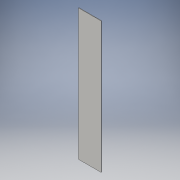
# Autodesk Inventor part: RightSidePlate
Saved by Autodesk Inventor 2016 (Build 200138000, 138)
## iProperties
Created: 2017-02-17
Part Number: RightSidePlate
Material: Generic
Document SubType Name: Modeling
Designer: RoboticsUser
Density: 1 g/cm^3
Appearance: Default
Author: RoboticsUser
Autodesk Inventor part; units mm, degrees
ref_plane "YZ Plane" through (0, 0, 0) normal (1, 0, 0) x (0, 1, 0)
ref_plane "XZ Plane" through (0, 0, 0) normal (0, 1, 0) x (-1, 0, 0)
ref_plane "XY Plane" through (0, 0, 0) normal (0, 0, 1) x (1, 0, 0)
sketch "Sketch1" plane through (0, 0, 0) normal (0, 0, 1) x (1, 0, 0)
  line L0 (0, 0) -> (76.2, 0)
  line L1 (76.2, 0) -> (76.2, 444.5)
  line L2 (76.2, 444.5) -> (0, 444.5)
  line L3 (0, 444.5) -> (0, 0)
  dimension "d0" = 76.2
  dimension "d1" = 444.5
  constraints: 8 end point, 2 parallel, 1 horizontal, 1 perpendicular
  measures "d0" distance of L2.end L1.end
  measures "d1" distance of L1.end L0.end
extrude "Extrusion1" add sketch "Sketch1" along normal blind 1.5875
body "Solid1"
